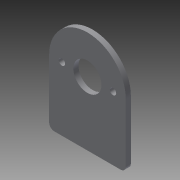
# Autodesk Inventor part: encoder_fixation
Saved by Autodesk Inventor 2014 SP1 (Build 180222100, 222)
## iProperties
Created: 2014-09-21
Part Number: encoder_fixation
Material: Générique
Document SubType Name: Modeling
Designer: astralien3000
Density: 1 g/cm^3
Appearance: Par défaut
d0: 30,000 mm
d1: 25,000 mm
d2: 2,000 mm
d3: 0,00 deg
d4: 2,500 mm
d5: 10,000 mm
d7: 0,00 deg
d8: 11,000 mm
d10: 0,00 deg
d11: 2,000 mm
Author: astralien3000
Autodesk Inventor part; units mm, degrees
ref_plane "YZ Plane" through (0, 0, 0) normal (1, 0, 0) x (0, 1, 0)
ref_plane "XZ Plane" through (0, 0, 0) normal (0, 1, 0) x (-1, 0, 0)
ref_plane "XY Plane" through (0, 0, 0) normal (0, 0, 1) x (1, 0, 0)
sketch "Esquisse1" plane through (0, 0, 0) normal (0, 1, 0) x (-1, 0, 0)
  arc A0 (15, 0) -> (-15, 0) centre (0, 0) ccw
  line L0 (-15, 0) -> (15, 0) construction
  line L1 (15, 0) -> (15, -25)
  line L2 (15, -25) -> (-15, -25)
  line L3 (-15, -25) -> (-15, 0)
  arc A1 (-15, 0) -> (15, 0) centre (0, 0) ccw construction
  dimension "d0" = 30
  dimension "d1" = 25
  constraints: 8 end point, 4 point on circle, 2 centre point, 2 parallel, 1 coincident, 1 horizontal, 1 midpoint, 1 perpendicular
  measures "d0" diameter of A0
  measures "d1" distance between parallel lines of L0 L2
extrude "Extrusion1" add sketch "Esquisse1" along normal blind 2
sketch "Esquisse2" plane through (0, 2, 0) normal (0, 1, 0) x (1, 0, 0)
  arc A0 (-15, 0) -> (15, 0) centre (0, 0) ccw projected
  line L0 (15, 25) -> (-15, 25) projected
  circle A1 centre (-10, 0) radius 1.25
  circle A2 centre (10, 0) radius 1.25
  line L1 (0, 0) -> (0, 25) construction
  line L2 (0, 0) -> (-15, 0) construction
  dimension "d4" = 2.5
  dimension "d5" = 10
  constraints: 4 end point, 2 centre point, 1 midpoint, 1 perpendicular, 1 point on line, 1 other
  measures "d4" diameter of A1
  measures "d5" distance from line of L1 A1.centre
extrude "Extrusion2" cut sketch "Esquisse2" against normal through all
sketch "Esquisse3" plane through (0, 2, 0) normal (0, 1, 0) x (1, 0, 0)
  arc A0 (-15, 0) -> (15, 0) centre (0, 0) ccw projected
  circle A1 centre (0, 0) radius 5.5
  dimension "d8" = 11
  constraints: 1 centre point, 1 coincident
  measures "d8" diameter of A1
extrude "Extrusion3" cut sketch "Esquisse3" against normal through all
fillet "Congé1" radius 2 2 edges at (-15, 1, -25) (15, 1, -25)
